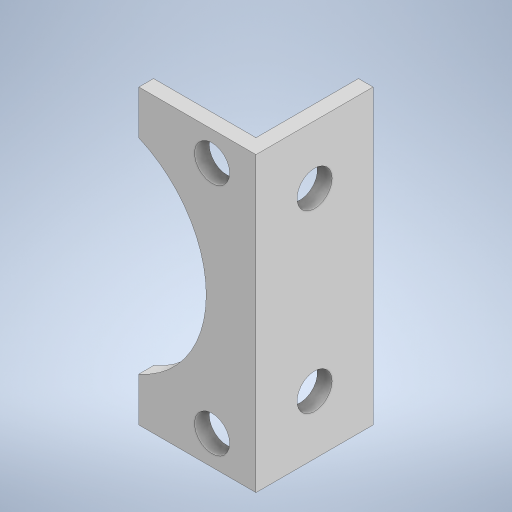
# Autodesk Inventor part: Cylinder Bracket
Saved by Autodesk Inventor 2023 (Build 270158000, 158)
## iProperties
Created: 2022-10-26
Part Number: Cylinder Bracket
Material: Generic
Document SubType Name: Modeling
Designer: tommy
Density: 1 g/cm^3
Appearance: Default
Author: tommy
Autodesk Inventor part; units mm, degrees
ref_plane "YZ Plane" through (0, 0, 0) normal (1, 0, 0) x (0, 1, 0)
ref_plane "XZ Plane" through (0, 0, 0) normal (0, 1, 0) x (-1, 0, 0)
ref_plane "XY Plane" through (0, 0, 0) normal (0, 0, 1) x (1, 0, 0)
sketch "Sketch1" plane through (0, 0, 0) normal (0, 1, 0) x (-1, 0, 0)
  line L0 (0, 0) -> (0, -25.4)
  line L1 (0, -25.4) -> (3.175, -25.4)
  line L2 (3.175, -25.4) -> (3.175, -3.175)
  line L3 (3.175, -3.175) -> (25.4, -3.175)
  line L4 (25.4, -3.175) -> (25.4, 0)
  line L5 (25.4, 0) -> (0, 0)
  dimension "d0" = 25.4
  dimension "d1" = 3.175
  dimension "d2" = 22.225
  dimension "d3" = 22.225
  constraints: 12 end point, 5 perpendicular, 1 vertical
  measures "d0" distance of L0.start L0.end
  measures "d1" distance of L0.end L1.end
  measures "d2" distance of L1.end L2.end
  measures "d3" distance of L2.end L3.end
extrude "Extrusion1" add sketch "Sketch1" along normal blind 63.5
sketch "Sketch2" plane through (-25.4, 0, 0) normal (0, 0, 1) x (1, 0, 0)
  line L0 (22.225, 0) -> (22.225, 63.5) projected
  line L1 (22.225, 0) -> (15.875, 0)
  line L2 (22.225, 0) -> (0, 0) projected
  line L3 (22.225, 63.5) -> (0, 63.5) projected
  circle A0 centre (15.875, 57.15) radius 3.81
  circle A1 centre (15.875, 6.35) radius 3.81
  circle A2 centre (-9.525, 31.75) radius 24.13
  line L4 (22.225, 31.75) -> (-9.525, 31.75)
  point P0 (25.4, 0)
  dimension "d6" = 6.35
  dimension "d9" = 7.62
  dimension "d10" = 7.62
  dimension "d12" = 31.75
  constraints: 4 end point, 3 centre point, 1 horizontal, 1 midpoint, 1 point on line
  measures "d6" distance of L0.start L1.end
  measures "d9" diameter of A0
  measures "d10" diameter of A1
  measures "d12" distance of L4.start L4.end
extrude "Extrusion2" cut sketch "Sketch2" against normal blind 63.5
sketch "Sketch3" plane through (0, 0, 0) normal (1, 0, 0) x (0, 0, -1)
  line L0 (25.4, 0) -> (25.4, 63.5) projected
  circle A0 centre (12.7, 12.7) radius 3.81
  line L1 (0, 9.5795) -> (0, 53.9205) projected
  circle A1 centre (12.7, 50.8) radius 3.81
  point P0 (0, 0)
  constraints: 2 centre point
extrude "Extrusion3" cut sketch "Sketch3" against normal blind 63.5
body "Solid1"
